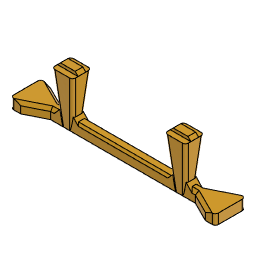
205mm Z Frame Spacer Jig v7 (Autodesk Fusion 360 design; units mm, degrees)
Autodesk Fusion 360 part; units mm, degrees
sketch "Sketch1" plane through (0, 0, 0) normal (0, 0, 1) x (1, 0, 0)
  line L0 (0, 0) -> (0, 30)
  line L1 (0, 30) -> (10, 30)
  line L2 (10, 30) -> (30, 20)
  line L3 (30, 20) -> (175, 20)
  line L4 (175, 20) -> (195, 30)
  line L5 (195, 30) -> (205, 30)
  line L6 (205, 30) -> (205, 0)
  line L7 (0, 15) -> (205, 15) construction
  line L8 (30, 10) -> (175, 10)
  line L9 (175, 10) -> (195, 0)
  line L10 (10, 0) -> (30, 10)
  line L11 (0, 0) -> (10, 0)
  line L12 (195, 0) -> (205, 0)
  dimension "d1" = 205
  dimension "d2" = 10
  dimension "d3" = 30
  dimension "d4" = 10
  dimension "d10" = 30
  constraint coincident L0.start L11.start
  constraint vertical L0
  constraint perpendicular L0 L1
  constraint parallel L1 L3
  constraint parallel L1 L5
  constraint perpendicular L5 L6
  constraint midpoint L0 L7.start
  constraint midpoint L6 L7.end
  constraint symmetric L0.end L7 L0.start
  constraint symmetric L1.end L7 L10.start
  constraint symmetric L2.end L7 L8.start
  constraint symmetric L3.end L7 L8.end
  constraint symmetric L4.end L7 L9.end
  constraint symmetric L5.end L7 L6.end
  constraint equal L1 L5
  constraint collinear L1 L5
  constraint horizontal L11
  constraint equal L2 L4
  measures "d1" distance of L0 L6
  measures "d2" distance of L0.end L1.end
  measures "d3" distance of L1 L11
  measures "d4" distance of L3 L8
  measures "d10" distance of L0 L2.end
extrude "Extrude1" add sketch "Sketch1" along normal blind 10
sketch "Sketch2" plane through (0, 0, 10) normal (0, 0, 1) x (-1, 0, 0)
  line L0 (0, 0) -> (-10, 0)
  line L1 (-10, 0) -> (-30, -10)
  line L2 (-30, -10) -> (-175, -10)
  line L3 (-175, -10) -> (-195, 0)
  line L4 (-195, 0) -> (-205, 0)
  line L5 (-205, 0) -> (-205, -30)
  line L6 (-205, -30) -> (-195, -30)
  line L7 (-195, -30) -> (-175, -20)
  line L8 (-175, -20) -> (-30, -20)
  line L9 (-30, -20) -> (-10, -30)
  line L10 (-10, -30) -> (0, -30)
  line L11 (0, -30) -> (0, 0)
  line L12 (-40, -20) -> (-52, -20)
  line L13 (-52, -20) -> (-52, -10)
  line L14 (-52, -10) -> (-40, -10)
  line L15 (-40, -10) -> (-40, -20)
  line L16 (-102.5, -20) -> (-102.5, 9.0965) construction
  line L17 (-165, -20) -> (-153, -20)
  line L18 (-153, -20) -> (-153, -10)
  line L19 (-153, -10) -> (-165, -10)
  line L20 (-165, -10) -> (-165, -20)
  dimension "d11" = 40
  dimension "d12" = 12
  constraint horizontal L12
  constraint vertical L13
  constraint horizontal L14
  constraint vertical L15
  constraint coincident L2 L13.end
  constraint coincident L8 L12.start
  constraint midpoint L8 L16.start
  constraint perpendicular L2 L16
  constraint symmetric L12.start L16 L17.start
  constraint symmetric L12.end L16 L17.end
  constraint symmetric L13.end L16 L18.end
  constraint symmetric L14.end L16 L19.end
  measures "d11" distance of L11 L15
  measures "d12" distance of L12.start L12.end
extrude "Extrude2" add sketch "Sketch2" along normal blind 50 draft 5 from surface at -10 contours L2 L8 L12 L13 L14 L15 | L2 L8 L17 L18 L19 L20
sketch "Sketch3" plane through (0, 0, 50) normal (0, 0, 1) x (-1, 0, 0)
  line L0 (-35.6256, -5.6256) -> (-56.3744, -5.6256)
  line L1 (-56.3744, -5.6256) -> (-56.3744, -24.3744)
  line L2 (-56.3744, -24.3744) -> (-35.6256, -24.3744)
  line L3 (-35.6256, -24.3744) -> (-35.6256, -5.6256)
  line L4 (-35.6256, -18.85) -> (-173.6141, -18.85)
  line L5 (-173.6141, -18.85) -> (-173.6141, -11.15)
  line L6 (-173.6141, -11.15) -> (-35.6256, -11.15)
  line L7 (-35.6256, -11.15) -> (-35.6256, -18.85)
  line L8 (-169.3744, -5.6256) -> (-169.3744, -24.3744)
  line L9 (-169.3744, -24.3744) -> (-148.6256, -24.3744)
  line L10 (-148.6256, -24.3744) -> (-148.6256, -5.6256)
  line L11 (-148.6256, -5.6256) -> (-169.3744, -5.6256)
  line L12 (-169.3744, -15) -> (9.765, -15) construction
  dimension "d16" = 7.7
  constraint horizontal L4
  constraint vertical L5
  constraint horizontal L6
  constraint vertical L7
  constraint coincident L3 L4.start
  constraint midpoint L8 L12.start
  constraint perpendicular L7 L12
  constraint symmetric L4 L6 L12
  measures "d16" distance of L4 L6
extrude "Extrude3" add sketch "Sketch3" along normal blind 3 contours L1 L3 L4 L6 L7 | L4 L6 L8 L10
chamfer "Chamfer1" distance 3 angle 45 12 edges at (34.5626, 10, 10) (170.4374, 10, 10) (170.4374, 20, 10) (34.5626, 20, 10) (20, 5, 10) (20, 25, 10) (185, 5, 10) (185, 25, 10) (39.1251, 15, 10) (52.8749, 15, 10) (152.1251, 15, 10) (165.8749, 15, 10)
fillet "Fillet1" radius 3 12 edges at (0, 0, 5) (0, 30, 5) (205, 30, 5) (205, 0, 5) (37.8128, 7.8128, 25) (54.1872, 7.8128, 25) (54.1872, 22.1872, 25) (37.8128, 22.1872, 25) (150.8128, 22.1872, 25) (167.1872, 22.1872, 25) (167.1872, 7.8128, 25) (150.8128, 7.8128, 25)
chamfer "Chamfer2" distance 3 angle 45 4 edges at (169.3744, 15, 53) (148.6256, 15, 53) (56.3744, 15, 53) (35.6256, 15, 53)
chamfer "Chamfer3" distance 2 angle 45 2 edges at (102.5, 10, 10) (102.5, 20, 10)
